Respeaker Spacer (Autodesk Fusion 360 design; units mm, degrees)
Autodesk Fusion 360 part; units mm, degrees
sketch "Sketch1" plane through (0, 0, 0) normal (0, 0, 1) x (1, 0, 0)
  line L0 (0, 0) -> (6, 0)
  line L1 (6, 0) -> (6, 6)
  line L2 (6, 6) -> (0, 6)
  line L3 (0, 6) -> (0, 0)
  line L4 (12, 0) -> (18, 0)
  line L5 (18, 0) -> (18, 6)
  line L6 (18, 6) -> (12, 6)
  line L7 (12, 6) -> (12, 0)
  line L8 (24, 0) -> (30, 0)
  line L9 (30, 0) -> (30, 6)
  line L10 (30, 6) -> (24, 6)
  line L11 (24, 6) -> (24, 0)
  line L12 (36, 0) -> (42, 0)
  line L13 (42, 0) -> (42, 6)
  line L14 (42, 6) -> (36, 6)
  line L15 (36, 6) -> (36, 0)
  line L16 (0, 0) -> (42, 0)
  line L17 (42, 0) -> (42, 6)
  line L18 (42, 6) -> (0, 6)
  line L19 (0, 6) -> (0, 0)
  circle A0 centre (3, 3) radius 1.25
  circle A1 centre (15, 3) radius 1.25
  circle A2 centre (27, 3) radius 1.25
  circle A3 centre (39, 3) radius 1.25
  dimension "d1" = 6
  dimension "d2" = 6
  dimension "d5" = 6
  dimension "d6" = 6
  dimension "d7" = 6
  dimension "d8" = 6
  dimension "d9" = 6
  dimension "d10" = 6
  dimension "d11" = 6
  dimension "d12" = 6
  dimension "d13" = 6
  dimension "d18" = 2.5
  dimension "d19" = 2.5
  dimension "d20" = 2.5
  dimension "d21" = 2.5
  constraint horizontal L0
  constraint vertical L1
  constraint horizontal L2
  constraint vertical L3
  constraint coincident L0.start L3.end
  constraint horizontal L4
  constraint vertical L5
  constraint horizontal L6
  constraint vertical L7
  constraint horizontal L8
  constraint vertical L9
  constraint horizontal L10
  constraint vertical L11
  constraint horizontal L12
  constraint vertical L13
  constraint horizontal L14
  constraint vertical L15
  constraint horizontal L16
  constraint vertical L17
  constraint horizontal L18
  constraint vertical L19
  measures "d1" distance of L0.start L0.end
  measures "d2" distance of L0.start L2.end
  measures "d5" distance of L4.start L4.end
  measures "d6" distance of L4.start L6.end
  measures "d7" distance of L8.start L8.end
  measures "d8" distance of L8.start L10.end
  measures "d9" distance of L12.start L14.end
  measures "d10" distance of L12.start L12.end
  measures "d11" distance of L0.end L4.start
  measures "d12" distance of L4.end L8.start
  measures "d13" distance of L8.end L12.start
  measures "d18" diameter of A0
  measures "d19" diameter of A1
  measures "d20" diameter of A2
  measures "d21" diameter of A3
extrude "Extrude2" add sketch "Sketch1" along normal blind 0.2 contours L0 L1 L2 L3 L16 L18 L19 | L1 L7 L16 L18 | L4 L5 L6 L7 L16 L18 | L5 L11 L16 L18 | L8 L9 L10 L11 L16 L18 | L9 L15 L16 L18 | L12 L13 L14 L15 L16 L17 L18 | A0 | A1 | A2 | A3
extrude "Extrude3" add sketch "Sketch1" along normal blind 3.7 contours L0 L1 L2 L3 L16 L18 L19 | L4 L5 L6 L7 L16 L18 | L8 L9 L10 L11 L16 L18 | L12 L13 L14 L15 L16 L17 L18 | A0 | A1 | A2 | A3
extrude "Extrude4" add sketch "Sketch1" along normal blind 5.7 contours A0 | A1 | A2 | A3
